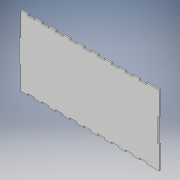
# Autodesk Inventor part: Pared2
Saved by Autodesk Inventor 2019 (Build 230136000, 136)
## iProperties
Created: 2020-03-08
Part Number: Pared2
Material: Genérico
Document SubType Name: Modeling
Designer: Diego Guillén
Density: 1 g/cm^3
Appearance: Valor por defecto
Author: Diego Guillén
Autodesk Inventor part; units mm, degrees
ref_plane "YZ Plane" through (0, 0, 0) normal (1, 0, 0) x (0, 1, 0)
ref_plane "XZ Plane" through (0, 0, 0) normal (0, 1, 0) x (-1, 0, 0)
ref_plane "XY Plane" through (0, 0, 0) normal (0, 0, 1) x (1, 0, 0)
sketch "Boceto1" plane through (0, 0, 0) normal (0, 0, 1) x (1, 0, 0)
  line L0 (0, 0) -> (300, 0)
  line L1 (300, 0) -> (300, 150)
  line L2 (300, 150) -> (0, 150)
  line L3 (0, 150) -> (0, 0)
  dimension "d0" = 150
  dimension "d1" = 300
  constraints: 8 end point, 2 parallel, 1 horizontal, 1 perpendicular
  measures "d0" distance of L0.end L1.end
  measures "d1" distance of L1.end L2.end
extrude "Extrusión1" add sketch "Boceto1" along normal blind 3
sketch "Boceto3" plane through (0, 0, 3) normal (0, 0, 1) x (1, 0, 0)
  line L0 (0, 0) -> (300, 0) construction
  line L1 (300, 0) -> (300, 150) construction
  line L2 (300, 150) -> (0, 150) construction
  line L3 (0, 150) -> (0, 0) construction
  line L4 (0, 50) -> (3, 50)
  line L5 (3, 50) -> (3, 0)
  line L6 (3, 0) -> (0, 0)
  line L7 (0, 0) -> (0, 50)
  line L8 (0, 100) -> (0, 150)
  line L9 (0, 150) -> (3, 150)
  line L10 (3, 150) -> (3, 100)
  line L11 (3, 100) -> (0, 100)
  line L12 (297, 100) -> (300, 100)
  line L13 (300, 100) -> (300, 50)
  line L14 (300, 50) -> (297, 50)
  line L15 (297, 50) -> (297, 100)
  line L16 (300, 0) -> (300, 150) construction
  point P0 (300, 75)
  point P1 (300, 75)
  dimension "d15" = 3
  dimension "d16" = 50
  dimension "d19" = 100
  dimension "d24" = 3
  dimension "d25" = 50
  constraints: 24 end point, 4 parallel, 2 coincident, 2 horizontal, 2 midpoint, 2 perpendicular, 1 collinear, 1 vertical, 8 other
  measures "d15" distance of L5.end L6.end
  measures "d16" distance of L4.end L5.end
  measures "d19" distance of L6.end L8.start
  measures "d24" distance of L13.end L14.end
  measures "d25" distance of L14.end L12.start
extrude "Extrusión3" cut sketch "Boceto3" against normal blind 3
sketch "Boceto4" plane through (0, 0, 3) normal (0, 0, 1) x (1, 0, 0)
  line L0 (3, 150) -> (3, 100) construction
  line L1 (3, 100) -> (0, 100) construction
  line L2 (0, 100) -> (0, 50) construction
  line L3 (0, 50) -> (3, 50) construction
  line L4 (3, 50) -> (3, 0) construction
  line L5 (3, 0) -> (300, 0) construction
  line L6 (300, 0) -> (300, 50) construction
  line L7 (300, 50) -> (297, 50) construction
  line L8 (297, 50) -> (297, 100) construction
  line L9 (297, 100) -> (300, 100) construction
  line L10 (300, 100) -> (300, 150) construction
  line L11 (300, 150) -> (3, 150) construction
  line L12 (18, 3) -> (33, 3)
  line L13 (33, 3) -> (33, 0)
  line L14 (33, 0) -> (18, 0)
  line L15 (18, 0) -> (18, 3)
  line L16 (18, 150) -> (33, 150)
  line L17 (33, 150) -> (33, 147)
  line L18 (33, 147) -> (18, 147)
  line L19 (18, 147) -> (18, 150)
  line L20 (300, 150) -> (3, 150) construction
  line L21 (3, 0) -> (300, 0) construction
  line L22 (48, 0) -> (48, 3)
  line L23 (63, 0) -> (48, 0)
  line L24 (48, 3) -> (63, 3)
  line L25 (63, 3) -> (63, 0)
  line L26 (48, 147) -> (48, 150)
  line L27 (48, 150) -> (63, 150)
  line L28 (63, 147) -> (48, 147)
  line L29 (63, 150) -> (63, 147)
  line L30 (78, 0) -> (78, 3)
  line L31 (93, 0) -> (78, 0)
  line L32 (78, 3) -> (93, 3)
  line L33 (93, 3) -> (93, 0)
  line L34 (78, 147) -> (78, 150)
  line L35 (78, 150) -> (93, 150)
  line L36 (93, 147) -> (78, 147)
  line L37 (93, 150) -> (93, 147)
  line L38 (108, 0) -> (108, 3)
  line L39 (123, 0) -> (108, 0)
  line L40 (108, 3) -> (123, 3)
  line L41 (123, 3) -> (123, 0)
  line L42 (108, 147) -> (108, 150)
  line L43 (108, 150) -> (123, 150)
  line L44 (123, 147) -> (108, 147)
  line L45 (123, 150) -> (123, 147)
  line L46 (138, 0) -> (138, 3)
  line L47 (153, 0) -> (138, 0)
  line L48 (138, 3) -> (153, 3)
  line L49 (153, 3) -> (153, 0)
  line L50 (138, 147) -> (138, 150)
  line L51 (138, 150) -> (153, 150)
  line L52 (153, 147) -> (138, 147)
  line L53 (153, 150) -> (153, 147)
  line L54 (168, 0) -> (168, 3)
  line L55 (183, 0) -> (168, 0)
  line L56 (168, 3) -> (183, 3)
  line L57 (183, 3) -> (183, 0)
  line L58 (168, 147) -> (168, 150)
  line L59 (168, 150) -> (183, 150)
  line L60 (183, 147) -> (168, 147)
  line L61 (183, 150) -> (183, 147)
  line L62 (198, 0) -> (198, 3)
  line L63 (213, 0) -> (198, 0)
  line L64 (198, 3) -> (213, 3)
  line L65 (213, 3) -> (213, 0)
  line L66 (198, 147) -> (198, 150)
  line L67 (198, 150) -> (213, 150)
  line L68 (213, 147) -> (198, 147)
  line L69 (213, 150) -> (213, 147)
  line L70 (228, 0) -> (228, 3)
  line L71 (243, 0) -> (228, 0)
  line L72 (228, 3) -> (243, 3)
  line L73 (243, 3) -> (243, 0)
  line L74 (228, 147) -> (228, 150)
  line L75 (228, 150) -> (243, 150)
  line L76 (243, 147) -> (228, 147)
  line L77 (243, 150) -> (243, 147)
  line L78 (258, 0) -> (258, 3)
  line L79 (273, 0) -> (258, 0)
  line L80 (258, 3) -> (273, 3)
  line L81 (273, 3) -> (273, 0)
  line L82 (258, 147) -> (258, 150)
  line L83 (258, 150) -> (273, 150)
  line L84 (273, 147) -> (258, 147)
  line L85 (273, 150) -> (273, 147)
  point P0 (0, 0)
  dimension "d28" = 3
  dimension "d29" = 3
  dimension "d30" = 15
  dimension "d31" = 15
  dimension "d32" = 15
  dimension "d33" = 15
  dimension "d36" = 30
  constraints: 144 end point, 4 parallel, 3 horizontal, 2 collinear, 2 perpendicular, 128 other
  measures "d28" distance of L16.end L17.end
  measures "d29" distance of L12.end L13.end
  measures "d30" distance of L17.end L18.end
  measures "d31" distance of L13.end L14.end
  measures "d32" distance between parallel lines of L4 L15
  measures "d33" distance between parallel lines of L0 L19
  measures "d36" distance of L14.end L22.start
extrude "Extrusión4" cut sketch "Boceto4" against normal blind 10
